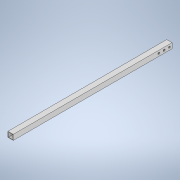
# Autodesk Inventor part: 3SR06_振子
Saved by Autodesk Inventor 2021 (Build 250183000, 183)
## iProperties
Created: 2021-04-20
Part Number: 3SR06_振子
Material: 一般
Document SubType Name: Modeling
Designer: ryusei
Density: 1 g/cm^3
Appearance: 既定
Author: ryusei
Autodesk Inventor part; units mm, degrees
ref_plane "YZ Plane" through (0, 0, 0) normal (1, 0, 0) x (0, 1, 0)
ref_plane "XZ Plane" through (0, 0, 0) normal (0, 1, 0) x (-1, 0, 0)
ref_plane "XY Plane" through (0, 0, 0) normal (0, 0, 1) x (1, 0, 0)
sketch "スケッチ1" plane through (0, 0, 0) normal (0, 0, 1) x (1, 0, 0)
  line L0 (0, 0) -> (10, 0)
  line L1 (10, 0) -> (10, 10)
  line L2 (10, 10) -> (0, 10)
  line L3 (0, 10) -> (0, 0)
  dimension "d0" = 10
  dimension "d1" = 10
  constraints: 8 end point, 2 parallel, 1 horizontal, 1 perpendicular
  measures "d0" distance between parallel lines of L0 L2
  measures "d1" distance between parallel lines of L1 L3
extrude "押し出し1" add sketch "スケッチ1" along normal blind 300
sketch "スケッチ2" plane through (0, 0, 300) normal (0, 0, 1) x (1, 0, 0)
  line L0 (1, 9) -> (9, 9)
  line L1 (9, 9) -> (9, 1)
  line L2 (9, 1) -> (1, 1)
  line L3 (1, 1) -> (1, 9)
  line L4 (10, 10) -> (0, 10) projected
  line L5 (10, 0) -> (10, 10) projected
  line L6 (0, 0) -> (10, 0) projected
  line L7 (0, 10) -> (0, 0) projected
  dimension "d4" = 1
  dimension "d5" = 1
  dimension "d6" = 1
  dimension "d7" = 1
  constraints: 8 end point, 2 parallel, 1 horizontal, 1 perpendicular
  measures "d4" distance between parallel lines of L4 L0
  measures "d5" distance between parallel lines of L5 L1
  measures "d6" distance between parallel lines of L6 L2
  measures "d7" distance between parallel lines of L7 L3
extrude "押し出し2" cut sketch "スケッチ2" against normal through all contours L0 L1 L2 L3
sketch "スケッチ3" plane through (10, 0, 0) normal (1, 0, 0) x (0, 0, -1)
  line L0 (0, 0) -> (0, 10) projected
  point P0 (-15, 5)
  dimension "d10" = 15
  measures "d10" distance from line of point (-15, 5) L0
hole "穴1" at (10, 5, 15) direction (-1, 0, 0) diameter 4 end through all
sketch "スケッチ4" plane through (10, 0, 0) normal (1, 0, 0) x (0, 0, -1)
  line L0 (0, 0) -> (0, 10) projected
  line L1 (0, 0) -> (-300, 0) projected
  point P0 (-5, 5)
  point P1 (-25, 5)
  dimension "d18" = 5
  dimension "d19" = 5
  dimension "d20" = 25
  measures "d18" distance from line of L0 point (-5, 5)
  measures "d19" distance from line of point (-5, 5) L1
  measures "d20" distance from line of L0 point (-25, 5)
hole "穴2" at (10, 5, 5) at (10, 5, 25) direction (-1, 0, 0) diameter 3.5 end through all
